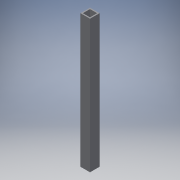
# Autodesk Inventor part: 15102898-16-P-0209
Saved by Autodesk Inventor 2017 (Build 210142000, 142)
## iProperties
Created: 2016-10-03
Part Number: 15102898-16-P-0209
Material: Aluminum 6061
Document SubType Name: Modeling
Designer: gus
Density: 2.7 g/cm^3
Appearance: Aluminum - Flat
Author: gus
Autodesk Inventor part; units mm, degrees
ref_plane "YZ Plane" through (0, 0, 0) normal (1, 0, 0) x (0, 1, 0)
ref_plane "XZ Plane" through (0, 0, 0) normal (0, 1, 0) x (-1, 0, 0)
ref_plane "XY Plane" through (0, 0, 0) normal (0, 0, 1) x (1, 0, 0)
sketch "Sketch1" plane through (0, 0, 0) normal (0, 1, 0) x (-1, 0, 0)
  line L0 (0, 0) -> (25.4, 0)
  line L1 (25.4, 0) -> (25.4, -25.4)
  line L2 (25.4, -25.4) -> (0, -25.4)
  line L3 (0, -25.4) -> (0, 0)
  line L4 (22.225, -22.225) -> (22.225, -3.175)
  line L5 (22.225, -3.175) -> (3.175, -3.175)
  line L6 (3.175, -3.175) -> (3.175, -22.225)
  line L7 (3.175, -22.225) -> (22.225, -22.225)
  dimension "d0" = 25.4
  dimension "d1" = 25.4
  dimension "d2" = 3.175
  constraints: 16 end point, 4 parallel, 2 perpendicular, 1 horizontal, 3 other
  measures "d0" distance of L1.end L2.end
  measures "d1" distance of L0.end L1.end
  measures "d2" distance between parallel lines of L1 L4
extrude "Extrusion1" add sketch "Sketch1" along normal blind 349.25
sketch "Sketch2" plane through (0, 0, 0) normal (1, 0, 0) x (0, 0, -1)
  line L0 (0, 0) -> (0, 349.25) projected
  line L1 (25.4, 0) -> (0, 0) projected
  line L2 (0, 349.25) -> (25.4, 349.25) projected
  point P0 (12.7, 12.7)
  point P1 (12.7, 38.1)
  point P2 (12.7, 336.55)
  point P3 (12.7, 311.15)
  dimension "d5" = 25.4
  dimension "d6" = 12.7
  dimension "d7" = 12.7
  dimension "d8" = 12.7
  dimension "d9" = 12.7
  dimension "d10" = 12.7
  dimension "d11" = 25.4
  dimension "d12" = 12.7
  measures "d5" distance of point (12.7, 311.15) point (12.7, 336.55)
  measures "d6" distance from line of L0 point (12.7, 336.55)
  measures "d7" distance from line of L0 point (12.7, 311.15)
  measures "d8" distance from line of L0 point (12.7, 38.1)
  measures "d9" distance from line of L0 point (12.7, 12.7)
  measures "d10" distance from line of L1 point (12.7, 12.7)
  measures "d11" distance of point (12.7, 12.7) point (12.7, 38.1)
  measures "d12" distance from line of L2 point (12.7, 336.55)
hole "Hole1" at (0, 12.7, -12.7) at (0, 38.1, -12.7) at (0, 336.55, -12.7) at (0, 311.15, -12.7) direction (-1, 0, 0) diameter 6.35 end through all
body "Solid1"
